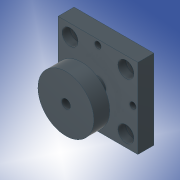
# Autodesk Inventor part: BA007
Saved by Autodesk Inventor 2017 SP1 (Build 210196100, 196)
## iProperties
Created: 2017-06-15
Part Number: BA007
Material: ABS Plastic
Document SubType Name: Modeling
Designer: zallen
Density: 1.06 g/cm^3
Appearance: CR Dark Blue
Author: zallen
Autodesk Inventor part; units mm, degrees
ref_plane "YZ Plane" through (0, 0, 0) normal (1, 0, 0) x (0, 1, 0)
ref_plane "XZ Plane" through (0, 0, 0) normal (0, 1, 0) x (-1, 0, 0)
ref_plane "XY Plane" through (0, 0, 0) normal (0, 0, 1) x (1, 0, 0)
sketch "Sketch1" plane through (0, 0, 0) normal (0, 0, 1) x (1, 0, 0)
  line L0 (0, 0) -> (50, 0)
  line L1 (50, 0) -> (50, 50)
  line L2 (50, 50) -> (0, 50)
  line L3 (0, 50) -> (0, 0)
  dimension "d0" = 50
  dimension "d1" = 50
  constraints: 8 end point, 2 parallel, 1 horizontal, 1 perpendicular
  measures "d0" distance of L2.end L1.end
  measures "d1" distance of L1.end L0.end
extrude "Extrusion1" add sketch "Sketch1" along normal blind 10
sketch "Sketch2" plane through (0, 0, 10) normal (0, 0, 1) x (1, 0, 0)
  line L0 (0, 50) -> (0, 0) construction
  line L1 (0, 25) -> (50, 25) construction
  line L2 (50, 0) -> (50, 50) construction
  line L3 (50, 50) -> (0, 50) construction
  line L4 (25, 50) -> (25, 0) construction
  line L5 (0, 0) -> (50, 0) construction
  line L6 (7.5, 7.5) -> (42.5, 7.5) construction
  line L7 (42.5, 7.5) -> (42.5, 42.5) construction
  line L8 (42.5, 42.5) -> (7.5, 42.5) construction
  line L9 (7.5, 42.5) -> (7.5, 7.5) construction
  line L10 (7.5, 7.5) -> (42.5, 42.5) construction
  line L11 (42.5, 7.5) -> (7.5, 42.5) construction
  circle A0 centre (42.5, 42.5) radius 2.5
  circle A1 centre (42.5, 7.5) radius 2.5
  circle A2 centre (7.5, 7.5) radius 2.5
  circle A3 centre (7.5, 42.5) radius 2.5
  point P0 (25, 25)
  dimension "d4" = 35
  dimension "d5" = 35
  dimension "d6" = 5
  dimension "d7" = 5
  dimension "d8" = 5
  dimension "d9" = 5
  constraints: 16 end point, 8 midpoint, 4 centre point, 4 coincident, 2 horizontal, 2 parallel, 1 perpendicular, 1 vertical
  measures "d4" distance of L8.end L7.end
  measures "d5" distance of L7.end L6.end
  measures "d6" diameter of A0
  measures "d7" diameter of A1
  measures "d8" diameter of A2
  measures "d9" diameter of A3
extrude "Extrusion2" cut sketch "Sketch2" against normal through all
sketch "Sketch3" plane through (0, 0, 10) normal (0, 0, 1) x (1, 0, 0)
  circle A0 centre (25, 25) radius 5
  line L0 (0, 50) -> (0, 0) projected
  line L1 (50, 50) -> (0, 50) projected
  point P0 (0, 25)
  point P1 (25, 50)
  dimension "d12" = 10
  constraints: 2 midpoint, 1 centre point, 1 horizontal alignment, 1 vertical alignment
  measures "d12" diameter of A0
extrude "Extrusion3" add sketch "Sketch3" along normal blind 10
sketch "Sketch4" plane through (25, 25, 20) normal (0, 0, 1) x (1, 0, 0)
  circle A0 centre (-0.1176, 0.006) radius 17.5
  arc A1 (17.3023, -1.6669) -> (17.3023, 1.679) centre (-0.1176, 0.006) ccw
  point P0 (-25, -25)
  dimension "d15" = 35
  constraints: 4 point on circle, 2 centre point, 1 concentric
  measures "d15" diameter of A0
extrude "Extrusion4" add sketch "Sketch4" along normal blind 10
sketch "Sketch5" plane through (0, 0, 10) normal (0, 0, 1) x (1, 0, 0)
  circle A0 centre (25, 25) radius 5 projected
  circle A1 centre (7.5, 7.5) radius 2.5 projected
  circle A2 centre (42.5, 42.5) radius 2.5 projected
  circle A3 centre (42.5, 7.5) radius 2.5 projected
  circle A4 centre (7.5, 42.5) radius 2.5 projected
  line L0 (0, 0) -> (50, 0) projected
  line L1 (50, 0) -> (50, 50) projected
  line L2 (50, 50) -> (0, 50) projected
  line L3 (0, 50) -> (0, 0) projected
  circle A5 centre (7.5, 42.5) radius 5
  circle A6 centre (42.5, 42.5) radius 5
  circle A7 centre (42.5, 7.5) radius 5
  circle A8 centre (7.5, 7.5) radius 2.5 projected
  circle A9 centre (7.5, 7.5) radius 5
  dimension "d28" = 10
  dimension "d29" = 10
  dimension "d30" = 10
  dimension "d31" = 10
  constraints: 4 centre point, 4 coincident
  measures "d28" diameter of A5
  measures "d29" diameter of A6
  measures "d30" diameter of A7
  measures "d31" diameter of A9
extrude "Extrusion5" cut sketch "Sketch5" against normal blind 5 contours A5 | A6 | A7 | A9
sketch "Sketch6" plane through (25, 25, 30) normal (0, 0, 1) x (1, 0, 0)
  circle A0 centre (0, 0) radius 2.75
  point P0 (-25, -25)
  dimension "d34" = 5.5
  constraints: 1 centre point
  measures "d34" diameter of A0
extrude "Extrusion6" cut sketch "Sketch6" against normal through all
sketch "Sketch7" plane through (0, 0, 0) normal (0, 0, -1) x (-1, 0, 0)
  circle A0 centre (-25, 25) radius 2.75 construction
  line L0 (-46.9203, 25) -> (-25, 46.9203) construction
  line L1 (-25, 46.9203) -> (-3.0797, 25) construction
  line L2 (-3.0797, 25) -> (-25, 3.0797) construction
  line L3 (-25, 3.0797) -> (-46.9203, 25) construction
  circle A1 centre (-25, 25) radius 5 construction
  line L4 (-46.9203, 25) -> (-3.0797, 25) construction
  line L5 (-25, 46.9203) -> (-25, 3.0797) construction
  line L6 (-46.9203, 25) -> (-15.9203, 25) construction
  circle A2 centre (-25, 46.9203) radius 2
  circle A3 centre (-3.0797, 25) radius 2
  circle A4 centre (-25, 3.0797) radius 2
  circle A5 centre (-46.9203, 25) radius 2
  dimension "d43" = 31
  dimension "d44" = 45
  dimension "d45" = 31
  dimension "d46" = 4
  dimension "d47" = 4
  dimension "d48" = 4
  dimension "d49" = 4
  constraints: 14 end point, 4 centre point, 4 coincident, 2 midpoint, 2 parallel, 1 equal length, 1 horizontal, 1 perpendicular
  measures "d43" distance of L0.start L0.end
  measures "d44" angle of L6 L0
  measures "d45" distance of L0.end L1.end
  measures "d46" diameter of A2
  measures "d47" diameter of A3
  measures "d48" diameter of A4
  measures "d49" diameter of A5
extrude "Extrusion7" cut sketch "Sketch7" against normal through all
body "Solid1"
